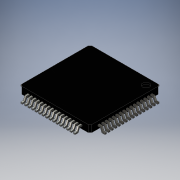
# Autodesk Inventor part: PIC16LF1946
Saved by Autodesk Inventor 2016 (Build 200138000, 138)
## iProperties
Created: 2016-08-10
Part Number: PIC16LF1946
Material: Generic
Document SubType Name: Modeling
Designer: jfixelle
Density: 1 g/cm^3
Appearance: Black
Author: jfixelle
## iProperties of the stored document PIC16LF1946_3DPrint.ipt
Created: 2016-08-10
Part Number: PIC16LF1946_3DPrint
Material: Generic
Document SubType Name: Modeling
Designer: jfixelle
Density: 1 g/cm^3
Appearance: Default
Author: jfixelle
Autodesk Inventor part; units mm, degrees
ref_plane "YZ Plane" through (0, 0, 0) normal (1, 0, 0) x (0, 1, 0)
sketch "Sketch1" plane through (0, 0, 0) normal (0, 1, 0) x (-1, 0, 0)
  line L0 (5, 5) -> (-5, 5)
  line L1 (-5, 5) -> (-5, -5)
  line L2 (-5, -5) -> (5, -5)
  line L3 (5, -5) -> (5, 5)
  circle A0 centre (-4, -4) radius 0.5
  point P0 (0, 0)
  dimension "d0" = 10
  dimension "d1" = 10
  dimension "d2" = 5
  dimension "d3" = 5
  dimension "d9" = 4
  dimension "d10" = 4
  dimension "d11" = 1
  constraints: 8 end point, 2 parallel, 1 centre point, 1 horizontal, 1 perpendicular
  measures "d0" distance of L2.end L0.start
  measures "d1" distance of L1.end L2.end
  measures "d2" distance from line of point (0, 0) L3
  measures "d3" distance from line of point (0, 0) L2
  measures "d9" horizontal distance of point (0, 0) A0.centre
  measures "d10" horizontal distance of point (0, 0) A0.centre
  measures "d11" diameter of A0
extrude "Extrusion1" add sketch "Sketch1" along normal blind 1 contours L3 L2 L1 L0 | A0
chamfer "Chamfer1" distance 0.25 angle 45 4 edges at (5, 0.5, 5) (5, 0.5, -5) (-5, 0.5, 5) (-5, 0.5, -5)
sketch "Sketch2" plane through (0, 1, 0) normal (0, 1, 0) x (1, 0, 0)
  circle A0 centre (4, 4) radius 0.5
  point P0 (0, 0)
  dimension "d12" = 1
  dimension "d13" = 4
  dimension "d14" = 4
  constraints: 1 centre point
  measures "d12" diameter of A0
  measures "d13" horizontal distance of point (0, 0) A0.centre
  measures "d14" horizontal distance of A0.centre point (0, 0)
extrude "Extrusion2" cut sketch "Sketch2" against normal blind 0.25
ref_plane "Work Plane3" through (3.75, 0, 4.75) normal (1, 0, 0) x (0, 0, -1)
sketch "Sketch7" plane through (3.75, 0, 4.75) normal (1, 0, 0) x (0, 0, -1)
  line L0 (-1.2492, -0.1997) -> (-0.7992, -0.1997)
  line L1 (-0.7992, -0.1997) -> (-0.5792, 0.3503)
  line L2 (-0.5792, 0.3503) -> (-0.2492, 0.3503)
  line L3 (-0.2492, 0.3503) -> (-0.2492, 0.5503)
  line L4 (-0.2492, 0.5503) -> (-0.6992, 0.5503)
  line L5 (-0.6992, 0.5503) -> (-0.9192, 0.0003)
  line L6 (-0.9192, 0.0003) -> (-1.2492, 0.0003)
  line L7 (-1.2492, 0.0003) -> (-1.2492, -0.1997)
  line L8 (-0.2492, 1.0003) -> (-0.2492, 0.0003)
  point P0 (4.75, 0)
  dimension "d40" = 0.2
  dimension "d41" = 0.2
  dimension "d42" = 1
  dimension "d43" = 0.75
  dimension "d44" = 0.45
  dimension "d45" = 0.33
  dimension "d46" = 0.45
  dimension "d47" = 0.33
  constraints: 18 end point, 3 perpendicular, 2 parallel
  measures "d40" distance of L6.end L0.start
  measures "d41" distance of L2.end L3.end
  measures "d42" distance between parallel lines of L3 L7
  measures "d43" distance between parallel lines of L4 L0
  measures "d44" distance of L0.start L0.end
  measures "d45" distance of L1.end L2.end
  measures "d46" distance of L3.end L4.end
  measures "d47" distance of L5.end L6.end
extrude "Extrusion4" add sketch "Sketch7" along normal mid plane 0.22
ref_plane "Work Plane4" through (-3.75, 0, 4.75) normal (1, 0, 0) x (0, 0, -1)
pattern_linear "Rectangular Pattern1" count 16 spacing 0.5 along (-1, 0, 0) of "Extrusion4"
mirror "Mirror1" about plane through (0, 0, 0) normal (0, 0, 1) of "Extrusion4", "Rectangular Pattern1"
pattern_circular "Circular Pattern1" count 2 over 90 about axis through (0, -10, 0) along (0, 1, 0) of "Extrusion4", "Rectangular Pattern1", "Mirror1"
ref_plane "Work Plane5" through (4.75, 0, 3.75) normal (0, 0, -1) x (-1, 0, 0)
body "Solid1"
